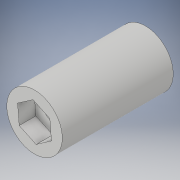
# Autodesk Inventor part: Vertical Sedder motor and rail coupler
Saved by Autodesk Inventor 2017 (Build 210142000, 142)
## iProperties
Created: 2017-05-24
Part Number: Vertical Sedder motor and rail coupler
Material: Generic
Document SubType Name: Modeling
Designer: Jon
Density: 1 g/cm^3
Appearance: Default
Author: Jon
Autodesk Inventor part; units mm, degrees
ref_plane "YZ Plane" through (0, 0, 0) normal (1, 0, 0) x (0, 1, 0)
ref_plane "XZ Plane" through (0, 0, 0) normal (0, 1, 0) x (-1, 0, 0)
ref_plane "XY Plane" through (0, 0, 0) normal (0, 0, 1) x (1, 0, 0)
sketch "Sketch3" plane through (0, 0, 0) normal (0, 0, 1) x (1, 0, 0)
  circle A0 centre (0, 0) radius 9.525
  dimension "d7" = 19.05
  constraints: 1 centre point, 1 coincident
  measures "d7" diameter of A0
extrude "Extrusion3" add sketch "Sketch3" along normal blind 38.1
sketch "Sketch4" plane through (0, 0, 38.1) normal (0, 0, 1) x (1, 0, 0)
  line L0 (5.2594, 3.6744) -> (5.8118, -2.7176)
  line L1 (5.8118, -2.7176) -> (0.5524, -6.392)
  line L2 (0.5524, -6.392) -> (-5.2594, -3.6744)
  line L3 (-5.2594, -3.6744) -> (-5.8118, 2.7176)
  line L4 (-5.8118, 2.7176) -> (-0.5524, 6.392)
  line L5 (-0.5524, 6.392) -> (5.2594, 3.6744)
  point P0 (0, 0)
  point P1 (0, 0)
  dimension "d10" = 11.1125
  constraints: 12 end point, 1 coincident, 13 other
  measures "d10" distance between parallel lines of L2 L5
extrude "Extrusion4" cut sketch "Sketch4" against normal blind 5.715
sketch "Sketch5" plane through (0, 0, 32.385) normal (0, 0, 1) x (1, 0, 0)
  circle A0 centre (0, 0) radius 2.3749
  dimension "d13" = 4.7498
  constraints: 1 centre point, 1 coincident
  measures "d13" diameter of A0
hole "Hole1" at (0, 0, 32.385) direction (0, 0, -1) diameter 4.7498 depth 13.335 tip angle 118
sketch "Sketch6" plane through (0, 0, 0) normal (0, 0, -1) x (-1, 0, 0)
  point P0 (0, 0)
sketch "Sketch7" plane through (0, 0, 0) normal (0, 0, -1) x (-1, 0, 0)
  point P0 (0, 0)
sketch "Sketch8" plane through (0, 0, 0) normal (0, 0, -1) x (-1, 0, 0)
  arc A0 (-1.6801, 1.905) -> (1.6801, 1.905) centre (0, 0) ccw
  line L0 (-1.6801, 1.905) -> (1.6801, 1.905)
  dimension "d21" = 5.08
  constraints: 2 end point, 2 point on circle, 1 centre point, 1 coincident, 1 horizontal
  measures "d21" diameter of A0
extrude "Extrusion5" cut sketch "Sketch8" against normal blind 19.05
body "Solid2"
